Autodesk Fusion 360 part; units mm, degrees
(part 2 of 2)
  line L726 (5.1001, -37.5652) -> (5.1001, -35.2552)
  line L727 (5.1001, -35.2552) -> (3.0996, -34.1002)
  line L728 (3.0996, -25.0042) -> (1.099, -26.1592)
  line L729 (1.099, -26.1592) -> (1.099, -28.4692)
  line L730 (1.099, -28.4692) -> (3.0996, -29.6242)
  line L731 (3.0996, -29.6242) -> (5.1001, -28.4692)
  line L732 (5.1001, -28.4692) -> (5.1001, -26.1592)
  line L733 (5.1001, -26.1592) -> (3.0996, -25.0042)
  line L734 (-2.0204, -34.1002) -> (-4.021, -35.2552)
  line L735 (-4.021, -35.2552) -> (-4.021, -37.5652)
  line L736 (-4.021, -37.5652) -> (-2.0204, -38.7202)
  line L737 (-2.0204, -38.7202) -> (-0.0199, -37.5652)
  line L738 (-0.0199, -37.5652) -> (-0.0199, -35.2552)
  line L739 (-0.0199, -35.2552) -> (-2.0204, -34.1002)
  line L740 (-2.0204, -25.0042) -> (-4.021, -26.1592)
  line L741 (-4.021, -26.1592) -> (-4.021, -28.4692)
  line L742 (-4.021, -28.4692) -> (-2.0204, -29.6242)
  line L743 (-2.0204, -29.6242) -> (-0.0199, -28.4692)
  line L744 (-0.0199, -28.4692) -> (-0.0199, -26.1592)
  line L745 (-0.0199, -26.1592) -> (-2.0204, -25.0042)
  line L746 (-7.1404, -34.1002) -> (-9.141, -35.2552)
  line L747 (-9.141, -35.2552) -> (-9.141, -37.5652)
  line L748 (-9.141, -37.5652) -> (-7.1404, -38.7202)
  line L749 (-7.1404, -38.7202) -> (-5.1399, -37.5652)
  line L750 (-5.1399, -37.5652) -> (-5.1399, -35.2552)
  line L751 (-5.1399, -35.2552) -> (-7.1404, -34.1002)
  line L752 (-7.1404, -25.0042) -> (-9.141, -26.1592)
  line L753 (-9.141, -26.1592) -> (-9.141, -28.4692)
  line L754 (-9.141, -28.4692) -> (-7.1404, -29.6242)
  line L755 (-7.1404, -29.6242) -> (-5.1399, -28.4692)
  line L756 (-5.1399, -28.4692) -> (-5.1399, -26.1592)
  line L757 (-5.1399, -26.1592) -> (-7.1404, -25.0042)
  line L758 (-12.2604, -34.1002) -> (-14.261, -35.2552)
  line L759 (-14.261, -35.2552) -> (-14.261, -37.5652)
  line L760 (-14.261, -37.5652) -> (-12.2604, -38.7202)
  line L761 (-12.2604, -38.7202) -> (-10.2599, -37.5652)
  line L762 (-10.2599, -37.5652) -> (-10.2599, -35.2552)
  line L763 (-10.2599, -35.2552) -> (-12.2604, -34.1002)
  line L764 (-12.2604, -25.0042) -> (-14.261, -26.1592)
  line L765 (-14.261, -26.1592) -> (-14.261, -28.4692)
  line L766 (-14.261, -28.4692) -> (-12.2604, -29.6242)
  line L767 (-12.2604, -29.6242) -> (-10.2599, -28.4692)
  line L768 (-10.2599, -28.4692) -> (-10.2599, -26.1592)
  line L769 (-10.2599, -26.1592) -> (-12.2604, -25.0042)
  line L770 (-17.3804, -34.1002) -> (-19.381, -35.2552)
  line L771 (-19.381, -35.2552) -> (-19.381, -37.5652)
  line L772 (-19.381, -37.5652) -> (-17.3804, -38.7202)
  line L773 (-17.3804, -38.7202) -> (-15.3799, -37.5652)
  line L774 (-15.3799, -37.5652) -> (-15.3799, -35.2552)
  line L775 (-15.3799, -35.2552) -> (-17.3804, -34.1002)
  line L776 (-17.3804, -25.0042) -> (-19.381, -26.1592)
  line L777 (-19.381, -26.1592) -> (-19.381, -28.4692)
  line L778 (-19.381, -28.4692) -> (-17.3804, -29.6242)
  line L779 (-17.3804, -29.6242) -> (-15.3799, -28.4692)
  line L780 (-15.3799, -28.4692) -> (-15.3799, -26.1592)
  line L781 (-15.3799, -26.1592) -> (-17.3804, -25.0042)
  line L782 (13.8344, 32.9648) -> (13.8344, 30.6548)
  line L783 (13.8344, 30.6548) -> (15.8349, 29.4998)
  line L784 (15.8349, 29.4998) -> (17.8354, 30.6548)
  line L785 (17.8354, 30.6548) -> (17.8354, 32.9648)
  line L786 (17.8354, 32.9648) -> (15.8349, 34.1198)
  line L787 (15.8349, 34.1198) -> (13.8344, 32.9648)
  line L788 (17.8354, 23.8688) -> (15.8349, 25.0238)
  line L789 (15.8349, 25.0238) -> (13.8344, 23.8688)
  line L790 (13.8344, 23.8688) -> (13.8344, 21.5588)
  line L791 (13.8344, 21.5588) -> (15.8349, 20.4038)
  line L792 (15.8349, 20.4038) -> (17.8354, 21.5588)
  line L793 (17.8354, 21.5588) -> (17.8354, 23.8688)
  line L794 (17.8354, 14.7728) -> (15.8349, 15.9278)
  line L795 (15.8349, 15.9278) -> (13.8344, 14.7728)
  line L796 (13.8344, 14.7728) -> (13.8344, 12.4628)
  line L797 (13.8344, 12.4628) -> (15.8349, 11.3078)
  line L798 (15.8349, 11.3078) -> (17.8354, 12.4628)
  line L799 (17.8354, 12.4628) -> (17.8354, 14.7728)
  line L800 (17.8354, 5.6768) -> (15.8349, 6.8318)
  line L801 (15.8349, 6.8318) -> (13.8344, 5.6768)
  line L802 (13.8344, 5.6768) -> (13.8344, 3.3668)
  line L803 (13.8344, 3.3668) -> (15.8349, 2.2118)
  line L804 (15.8349, 2.2118) -> (17.8354, 3.3668)
  line L805 (17.8354, 3.3668) -> (17.8354, 5.6768)
  line L806 (17.8354, -3.4192) -> (15.8349, -2.2642)
  line L807 (15.8349, -2.2642) -> (13.8344, -3.4192)
  line L808 (13.8344, -3.4192) -> (13.8344, -5.7292)
  line L809 (13.8344, -5.7292) -> (15.8349, -6.8842)
  line L810 (15.8349, -6.8842) -> (17.8354, -5.7292)
  line L811 (17.8354, -5.7292) -> (17.8354, -3.4192)
  line L812 (17.8354, -12.5152) -> (15.8349, -11.3602)
  line L813 (15.8349, -11.3602) -> (13.8344, -12.5152)
  line L814 (13.8344, -12.5152) -> (13.8344, -14.8252)
  line L815 (13.8344, -14.8252) -> (15.8349, -15.9802)
  line L816 (15.8349, -15.9802) -> (17.8354, -14.8252)
  line L817 (17.8354, -14.8252) -> (17.8354, -12.5152)
  line L818 (17.8354, -21.6112) -> (15.8349, -20.4562)
  line L819 (15.8349, -20.4562) -> (13.8344, -21.6112)
  line L820 (13.8344, -21.6112) -> (13.8344, -23.9212)
  line L821 (13.8344, -23.9212) -> (15.8349, -25.0762)
  line L822 (15.8349, -25.0762) -> (17.8354, -23.9212)
  line L823 (17.8354, -23.9212) -> (17.8354, -21.6112)
  line L824 (17.8354, -30.7072) -> (15.8349, -29.5522)
  line L825 (15.8349, -29.5522) -> (13.8344, -30.7072)
  line L826 (13.8344, -30.7072) -> (13.8344, -33.0172)
  line L827 (13.8344, -33.0172) -> (15.8349, -34.1722)
  line L828 (15.8349, -34.1722) -> (17.8354, -33.0172)
  line L829 (17.8354, -33.0172) -> (17.8354, -30.7072)
  line L830 (12.7154, 32.9648) -> (10.7149, 34.1198)
  line L831 (10.7149, 34.1198) -> (8.7144, 32.9648)
  line L832 (8.7144, 32.9648) -> (8.7144, 30.6548)
  line L833 (8.7144, 30.6548) -> (10.7149, 29.4998)
  line L834 (10.7149, 29.4998) -> (12.7154, 30.6548)
  line L835 (12.7154, 30.6548) -> (12.7154, 32.9648)
  line L836 (7.5954, 32.9648) -> (5.5949, 34.1198)
  line L837 (5.5949, 34.1198) -> (3.5944, 32.9648)
  line L838 (3.5944, 32.9648) -> (3.5944, 30.6548)
  line L839 (3.5944, 30.6548) -> (5.5949, 29.4998)
  line L840 (5.5949, 29.4998) -> (7.5954, 30.6548)
  line L841 (7.5954, 30.6548) -> (7.5954, 32.9648)
  line L842 (2.4754, 32.9648) -> (0.4749, 34.1198)
  line L843 (0.4749, 34.1198) -> (-1.5256, 32.9648)
  line L844 (-1.5256, 32.9648) -> (-1.5256, 30.6548)
  line L845 (-1.5256, 30.6548) -> (0.4749, 29.4998)
  line L846 (0.4749, 29.4998) -> (2.4754, 30.6548)
  line L847 (2.4754, 30.6548) -> (2.4754, 32.9648)
  line L848 (-2.6446, 32.9648) -> (-4.6451, 34.1198)
  line L849 (-4.6451, 34.1198) -> (-6.6456, 32.9648)
  line L850 (-6.6456, 32.9648) -> (-6.6456, 30.6548)
  line L851 (-6.6456, 30.6548) -> (-4.6451, 29.4998)
  line L852 (-4.6451, 29.4998) -> (-2.6446, 30.6548)
  line L853 (-2.6446, 30.6548) -> (-2.6446, 32.9648)
  line L854 (-7.7646, 32.9648) -> (-9.7651, 34.1198)
  line L855 (-9.7651, 34.1198) -> (-11.7656, 32.9648)
  line L856 (-11.7656, 32.9648) -> (-11.7656, 30.6548)
  line L857 (-11.7656, 30.6548) -> (-9.7651, 29.4998)
  line L858 (-9.7651, 29.4998) -> (-7.7646, 30.6548)
  line L859 (-7.7646, 30.6548) -> (-7.7646, 32.9648)
  line L860 (-12.8846, 32.9648) -> (-14.8851, 34.1198)
  line L861 (-14.8851, 34.1198) -> (-16.8856, 32.9648)
  line L862 (-16.8856, 32.9648) -> (-16.8856, 30.6548)
  line L863 (-16.8856, 30.6548) -> (-14.8851, 29.4998)
  line L864 (-14.8851, 29.4998) -> (-12.8846, 30.6548)
  line L865 (-12.8846, 30.6548) -> (-12.8846, 32.9648)
  line L866 (12.7154, 23.8688) -> (10.7149, 25.0238)
  line L867 (10.7149, 25.0238) -> (8.7144, 23.8688)
  line L868 (8.7144, 23.8688) -> (8.7144, 21.5588)
  line L869 (8.7144, 21.5588) -> (10.7149, 20.4038)
  line L870 (10.7149, 20.4038) -> (12.7154, 21.5588)
  line L871 (12.7154, 21.5588) -> (12.7154, 23.8688)
  line L872 (7.5954, 23.8688) -> (5.5949, 25.0238)
  line L873 (5.5949, 25.0238) -> (3.5944, 23.8688)
  line L874 (3.5944, 23.8688) -> (3.5944, 21.5588)
  line L875 (3.5944, 21.5588) -> (5.5949, 20.4038)
  line L876 (5.5949, 20.4038) -> (7.5954, 21.5588)
  line L877 (7.5954, 21.5588) -> (7.5954, 23.8688)
  line L878 (2.4754, 23.8688) -> (0.4749, 25.0238)
  line L879 (0.4749, 25.0238) -> (-1.5256, 23.8688)
  line L880 (-1.5256, 23.8688) -> (-1.5256, 21.5588)
  line L881 (-1.5256, 21.5588) -> (0.4749, 20.4038)
  line L882 (0.4749, 20.4038) -> (2.4754, 21.5588)
  line L883 (2.4754, 21.5588) -> (2.4754, 23.8688)
  line L884 (-2.6446, 23.8688) -> (-4.6451, 25.0238)
  line L885 (-4.6451, 25.0238) -> (-6.6456, 23.8688)
  line L886 (-6.6456, 23.8688) -> (-6.6456, 21.5588)
  line L887 (-6.6456, 21.5588) -> (-4.6451, 20.4038)
  line L888 (-4.6451, 20.4038) -> (-2.6446, 21.5588)
  line L889 (-2.6446, 21.5588) -> (-2.6446, 23.8688)
  line L890 (-7.7646, 23.8688) -> (-9.7651, 25.0238)
  line L891 (-9.7651, 25.0238) -> (-11.7656, 23.8688)
  line L892 (-11.7656, 23.8688) -> (-11.7656, 21.5588)
  line L893 (-11.7656, 21.5588) -> (-9.7651, 20.4038)
  line L894 (-9.7651, 20.4038) -> (-7.7646, 21.5588)
  line L895 (-7.7646, 21.5588) -> (-7.7646, 23.8688)
  line L896 (-12.8846, 23.8688) -> (-14.8851, 25.0238)
  line L897 (-14.8851, 25.0238) -> (-16.8856, 23.8688)
  line L898 (-16.8856, 23.8688) -> (-16.8856, 21.5588)
  line L899 (-16.8856, 21.5588) -> (-14.8851, 20.4038)
  line L900 (-14.8851, 20.4038) -> (-12.8846, 21.5588)
  line L901 (-12.8846, 21.5588) -> (-12.8846, 23.8688)
  line L902 (12.7154, 14.7728) -> (10.7149, 15.9278)
  line L903 (10.7149, 15.9278) -> (8.7144, 14.7728)
  line L904 (8.7144, 14.7728) -> (8.7144, 12.4628)
  line L905 (8.7144, 12.4628) -> (10.7149, 11.3078)
  line L906 (10.7149, 11.3078) -> (12.7154, 12.4628)
  line L907 (12.7154, 12.4628) -> (12.7154, 14.7728)
  line L908 (7.5954, 14.7728) -> (5.5949, 15.9278)
  line L909 (5.5949, 15.9278) -> (3.5944, 14.7728)
  line L910 (3.5944, 14.7728) -> (3.5944, 12.4628)
  line L911 (3.5944, 12.4628) -> (5.5949, 11.3078)
  line L912 (5.5949, 11.3078) -> (7.5954, 12.4628)
  line L913 (7.5954, 12.4628) -> (7.5954, 14.7728)
  line L914 (2.4754, 14.7728) -> (0.4749, 15.9278)
  line L915 (0.4749, 15.9278) -> (-1.5256, 14.7728)
  line L916 (-1.5256, 14.7728) -> (-1.5256, 12.4628)
  line L917 (-1.5256, 12.4628) -> (0.4749, 11.3078)
  line L918 (0.4749, 11.3078) -> (2.4754, 12.4628)
  line L919 (2.4754, 12.4628) -> (2.4754, 14.7728)
  line L920 (-2.6446, 14.7728) -> (-4.6451, 15.9278)
  line L921 (-4.6451, 15.9278) -> (-6.6456, 14.7728)
  line L922 (-6.6456, 14.7728) -> (-6.6456, 12.4628)
  line L923 (-6.6456, 12.4628) -> (-4.6451, 11.3078)
  line L924 (-4.6451, 11.3078) -> (-2.6446, 12.4628)
  line L925 (-2.6446, 12.4628) -> (-2.6446, 14.7728)
  line L926 (-7.7646, 14.7728) -> (-9.7651, 15.9278)
  line L927 (-9.7651, 15.9278) -> (-11.7656, 14.7728)
  line L928 (-11.7656, 14.7728) -> (-11.7656, 12.4628)
  line L929 (-11.7656, 12.4628) -> (-9.7651, 11.3078)
  line L930 (-9.7651, 11.3078) -> (-7.7646, 12.4628)
  line L931 (-7.7646, 12.4628) -> (-7.7646, 14.7728)
  line L932 (-12.8846, 14.7728) -> (-14.8851, 15.9278)
  line L933 (-14.8851, 15.9278) -> (-16.8856, 14.7728)
  line L934 (-16.8856, 14.7728) -> (-16.8856, 12.4628)
  line L935 (-16.8856, 12.4628) -> (-14.8851, 11.3078)
  line L936 (-14.8851, 11.3078) -> (-12.8846, 12.4628)
  line L937 (-12.8846, 12.4628) -> (-12.8846, 14.7728)
  line L938 (12.7154, 5.6768) -> (10.7149, 6.8318)
  line L939 (10.7149, 6.8318) -> (8.7144, 5.6768)
  line L940 (8.7144, 5.6768) -> (8.7144, 3.3668)
  line L941 (8.7144, 3.3668) -> (10.7149, 2.2118)
  line L942 (10.7149, 2.2118) -> (12.7154, 3.3668)
  line L943 (12.7154, 3.3668) -> (12.7154, 5.6768)
  line L944 (7.5954, 5.6768) -> (5.5949, 6.8318)
  line L945 (5.5949, 6.8318) -> (3.5944, 5.6768)
  line L946 (3.5944, 5.6768) -> (3.5944, 3.3668)
  line L947 (3.5944, 3.3668) -> (5.5949, 2.2118)
  line L948 (5.5949, 2.2118) -> (7.5954, 3.3668)
  line L949 (7.5954, 3.3668) -> (7.5954, 5.6768)
  line L950 (2.4754, 5.6768) -> (0.4749, 6.8318)
  line L951 (0.4749, 6.8318) -> (-1.5256, 5.6768)
  line L952 (-1.5256, 5.6768) -> (-1.5256, 3.3668)
  line L953 (-1.5256, 3.3668) -> (0.4749, 2.2118)
  line L954 (0.4749, 2.2118) -> (2.4754, 3.3668)
  line L955 (2.4754, 3.3668) -> (2.4754, 5.6768)
  line L956 (-2.6446, 5.6768) -> (-4.6451, 6.8318)
  line L957 (-4.6451, 6.8318) -> (-6.6456, 5.6768)
  line L958 (-6.6456, 5.6768) -> (-6.6456, 3.3668)
  line L959 (-6.6456, 3.3668) -> (-4.6451, 2.2118)
  line L960 (-4.6451, 2.2118) -> (-2.6446, 3.3668)
  line L961 (-2.6446, 3.3668) -> (-2.6446, 5.6768)
  line L962 (-7.7646, 5.6768) -> (-9.7651, 6.8318)
  line L963 (-9.7651, 6.8318) -> (-11.7656, 5.6768)
  line L964 (-11.7656, 5.6768) -> (-11.7656, 3.3668)
  line L965 (-11.7656, 3.3668) -> (-9.7651, 2.2118)
  line L966 (-9.7651, 2.2118) -> (-7.7646, 3.3668)
  line L967 (-7.7646, 3.3668) -> (-7.7646, 5.6768)
  line L968 (-12.8846, 5.6768) -> (-14.8851, 6.8318)
  line L969 (-14.8851, 6.8318) -> (-16.8856, 5.6768)
  line L970 (-16.8856, 5.6768) -> (-16.8856, 3.3668)
  line L971 (-16.8856, 3.3668) -> (-14.8851, 2.2118)
  line L972 (-14.8851, 2.2118) -> (-12.8846, 3.3668)
  line L973 (-12.8846, 3.3668) -> (-12.8846, 5.6768)
  line L974 (12.7154, -3.4192) -> (10.7149, -2.2642)
  line L975 (10.7149, -2.2642) -> (8.7144, -3.4192)
  line L976 (8.7144, -3.4192) -> (8.7144, -5.7292)
  line L977 (8.7144, -5.7292) -> (10.7149, -6.8842)
  line L978 (10.7149, -6.8842) -> (12.7154, -5.7292)
  line L979 (12.7154, -5.7292) -> (12.7154, -3.4192)
  line L980 (7.5954, -3.4192) -> (5.5949, -2.2642)
  line L981 (5.5949, -2.2642) -> (3.5944, -3.4192)
  line L982 (3.5944, -3.4192) -> (3.5944, -5.7292)
  line L983 (3.5944, -5.7292) -> (5.5949, -6.8842)
  line L984 (5.5949, -6.8842) -> (7.5954, -5.7292)
  line L985 (7.5954, -5.7292) -> (7.5954, -3.4192)
  line L986 (2.4754, -3.4192) -> (0.4749, -2.2642)
  line L987 (0.4749, -2.2642) -> (-1.5256, -3.4192)
  line L988 (-1.5256, -3.4192) -> (-1.5256, -5.7292)
  line L989 (-1.5256, -5.7292) -> (0.4749, -6.8842)
  line L990 (0.4749, -6.8842) -> (2.4754, -5.7292)
  line L991 (2.4754, -5.7292) -> (2.4754, -3.4192)
  line L992 (-2.6446, -3.4192) -> (-4.6451, -2.2642)
  line L993 (-4.6451, -2.2642) -> (-6.6456, -3.4192)
  line L994 (-6.6456, -3.4192) -> (-6.6456, -5.7292)
  line L995 (-6.6456, -5.7292) -> (-4.6451, -6.8842)
  line L996 (-4.6451, -6.8842) -> (-2.6446, -5.7292)
  line L997 (-2.6446, -5.7292) -> (-2.6446, -3.4192)
  line L998 (-7.7646, -3.4192) -> (-9.7651, -2.2642)
  line L999 (-9.7651, -2.2642) -> (-11.7656, -3.4192)
  line L1000 (-11.7656, -3.4192) -> (-11.7656, -5.7292)
  line L1001 (-11.7656, -5.7292) -> (-9.7651, -6.8842)
  line L1002 (-9.7651, -6.8842) -> (-7.7646, -5.7292)
  line L1003 (-7.7646, -5.7292) -> (-7.7646, -3.4192)
  line L1004 (-12.8846, -3.4192) -> (-14.8851, -2.2642)
  line L1005 (-14.8851, -2.2642) -> (-16.8856, -3.4192)
  line L1006 (-16.8856, -3.4192) -> (-16.8856, -5.7292)
  line L1007 (-16.8856, -5.7292) -> (-14.8851, -6.8842)
  line L1008 (-14.8851, -6.8842) -> (-12.8846, -5.7292)
  line L1009 (-12.8846, -5.7292) -> (-12.8846, -3.4192)
  line L1010 (12.7154, -12.5152) -> (10.7149, -11.3602)
  line L1011 (10.7149, -11.3602) -> (8.7144, -12.5152)
  line L1012 (8.7144, -12.5152) -> (8.7144, -14.8252)
  line L1013 (8.7144, -14.8252) -> (10.7149, -15.9802)
  line L1014 (10.7149, -15.9802) -> (12.7154, -14.8252)
  line L1015 (12.7154, -14.8252) -> (12.7154, -12.5152)
  line L1016 (7.5954, -12.5152) -> (5.5949, -11.3602)
  line L1017 (5.5949, -11.3602) -> (3.5944, -12.5152)
  line L1018 (3.5944, -12.5152) -> (3.5944, -14.8252)
  line L1019 (3.5944, -14.8252) -> (5.5949, -15.9802)
  line L1020 (5.5949, -15.9802) -> (7.5954, -14.8252)
  line L1021 (7.5954, -14.8252) -> (7.5954, -12.5152)
  line L1022 (2.4754, -12.5152) -> (0.4749, -11.3602)
  line L1023 (0.4749, -11.3602) -> (-1.5256, -12.5152)
  line L1024 (-1.5256, -12.5152) -> (-1.5256, -14.8252)
  line L1025 (-1.5256, -14.8252) -> (0.4749, -15.9802)
  line L1026 (0.4749, -15.9802) -> (2.4754, -14.8252)
  line L1027 (2.4754, -14.8252) -> (2.4754, -12.5152)
  line L1028 (-2.6446, -12.5152) -> (-4.6451, -11.3602)
  line L1029 (-4.6451, -11.3602) -> (-6.6456, -12.5152)
  line L1030 (-6.6456, -12.5152) -> (-6.6456, -14.8252)
  line L1031 (-6.6456, -14.8252) -> (-4.6451, -15.9802)
  line L1032 (-4.6451, -15.9802) -> (-2.6446, -14.8252)
  line L1033 (-2.6446, -14.8252) -> (-2.6446, -12.5152)
  line L1034 (-7.7646, -12.5152) -> (-9.7651, -11.3602)
  line L1035 (-9.7651, -11.3602) -> (-11.7656, -12.5152)
  line L1036 (-11.7656, -12.5152) -> (-11.7656, -14.8252)
  line L1037 (-11.7656, -14.8252) -> (-9.7651, -15.9802)
  line L1038 (-9.7651, -15.9802) -> (-7.7646, -14.8252)
  line L1039 (-7.7646, -14.8252) -> (-7.7646, -12.5152)
  line L1040 (-12.8846, -12.5152) -> (-14.8851, -11.3602)
  line L1041 (-14.8851, -11.3602) -> (-16.8856, -12.5152)
  line L1042 (-16.8856, -12.5152) -> (-16.8856, -14.8252)
  line L1043 (-16.8856, -14.8252) -> (-14.8851, -15.9802)
  line L1044 (-14.8851, -15.9802) -> (-12.8846, -14.8252)
  line L1045 (-12.8846, -14.8252) -> (-12.8846, -12.5152)
  line L1046 (12.7154, -21.6112) -> (10.7149, -20.4562)
  line L1047 (10.7149, -20.4562) -> (8.7144, -21.6112)
  line L1048 (8.7144, -21.6112) -> (8.7144, -23.9212)
  line L1049 (8.7144, -23.9212) -> (10.7149, -25.0762)
  line L1050 (10.7149, -25.0762) -> (12.7154, -23.9212)
  line L1051 (12.7154, -23.9212) -> (12.7154, -21.6112)
  line L1052 (7.5954, -21.6112) -> (5.5949, -20.4562)
  line L1053 (5.5949, -20.4562) -> (3.5944, -21.6112)
  line L1054 (3.5944, -21.6112) -> (3.5944, -23.9212)
  line L1055 (3.5944, -23.9212) -> (5.5949, -25.0762)
  line L1056 (5.5949, -25.0762) -> (7.5954, -23.9212)
  line L1057 (7.5954, -23.9212) -> (7.5954, -21.6112)
  line L1058 (2.4754, -21.6112) -> (0.4749, -20.4562)
  line L1059 (0.4749, -20.4562) -> (-1.5256, -21.6112)
  line L1060 (-1.5256, -21.6112) -> (-1.5256, -23.9212)
  line L1061 (-1.5256, -23.9212) -> (0.4749, -25.0762)
  line L1062 (0.4749, -25.0762) -> (2.4754, -23.9212)
  line L1063 (2.4754, -23.9212) -> (2.4754, -21.6112)
  line L1064 (-2.6446, -21.6112) -> (-4.6451, -20.4562)
  line L1065 (-4.6451, -20.4562) -> (-6.6456, -21.6112)
  line L1066 (-6.6456, -21.6112) -> (-6.6456, -23.9212)
  line L1067 (-6.6456, -23.9212) -> (-4.6451, -25.0762)
  line L1068 (-4.6451, -25.0762) -> (-2.6446, -23.9212)
  line L1069 (-2.6446, -23.9212) -> (-2.6446, -21.6112)
  line L1070 (-7.7646, -21.6112) -> (-9.7651, -20.4562)
  line L1071 (-9.7651, -20.4562) -> (-11.7656, -21.6112)
  line L1072 (-11.7656, -21.6112) -> (-11.7656, -23.9212)
  line L1073 (-11.7656, -23.9212) -> (-9.7651, -25.0762)
  line L1074 (-9.7651, -25.0762) -> (-7.7646, -23.9212)
  line L1075 (-7.7646, -23.9212) -> (-7.7646, -21.6112)
  line L1076 (-12.8846, -21.6112) -> (-14.8851, -20.4562)
  line L1077 (-14.8851, -20.4562) -> (-16.8856, -21.6112)
  line L1078 (-16.8856, -21.6112) -> (-16.8856, -23.9212)
  line L1079 (-16.8856, -23.9212) -> (-14.8851, -25.0762)
  line L1080 (-14.8851, -25.0762) -> (-12.8846, -23.9212)
  line L1081 (-12.8846, -23.9212) -> (-12.8846, -21.6112)
  line L1082 (12.7154, -30.7072) -> (10.7149, -29.5522)
  line L1083 (10.7149, -29.5522) -> (8.7144, -30.7072)
  line L1084 (8.7144, -30.7072) -> (8.7144, -33.0172)
  line L1085 (8.7144, -33.0172) -> (10.7149, -34.1722)
  line L1086 (10.7149, -34.1722) -> (12.7154, -33.0172)
  line L1087 (12.7154, -33.0172) -> (12.7154, -30.7072)
  line L1088 (7.5954, -30.7072) -> (5.5949, -29.5522)
  line L1089 (5.5949, -29.5522) -> (3.5944, -30.7072)
  line L1090 (3.5944, -30.7072) -> (3.5944, -33.0172)
  line L1091 (3.5944, -33.0172) -> (5.5949, -34.1722)
  line L1092 (5.5949, -34.1722) -> (7.5954, -33.0172)
  line L1093 (7.5954, -33.0172) -> (7.5954, -30.7072)
  line L1094 (2.4754, -30.7072) -> (0.4749, -29.5522)
  line L1095 (0.4749, -29.5522) -> (-1.5256, -30.7072)
  line L1096 (-1.5256, -30.7072) -> (-1.5256, -33.0172)
  line L1097 (-1.5256, -33.0172) -> (0.4749, -34.1722)
  line L1098 (0.4749, -34.1722) -> (2.4754, -33.0172)
  line L1099 (2.4754, -33.0172) -> (2.4754, -30.7072)
  line L1100 (-2.6446, -30.7072) -> (-4.6451, -29.5522)
  line L1101 (-4.6451, -29.5522) -> (-6.6456, -30.7072)
  line L1102 (-6.6456, -30.7072) -> (-6.6456, -33.0172)
  line L1103 (-6.6456, -33.0172) -> (-4.6451, -34.1722)
  line L1104 (-4.6451, -34.1722) -> (-2.6446, -33.0172)
  line L1105 (-2.6446, -33.0172) -> (-2.6446, -30.7072)
  line L1106 (-7.7646, -30.7072) -> (-9.7651, -29.5522)
  line L1107 (-9.7651, -29.5522) -> (-11.7656, -30.7072)
  line L1108 (-11.7656, -30.7072) -> (-11.7656, -33.0172)
  line L1109 (-11.7656, -33.0172) -> (-9.7651, -34.1722)
  line L1110 (-9.7651, -34.1722) -> (-7.7646, -33.0172)
  line L1111 (-7.7646, -33.0172) -> (-7.7646, -30.7072)
  line L1112 (-12.8846, -30.7072) -> (-14.8851, -29.5522)
  line L1113 (-14.8851, -29.5522) -> (-16.8856, -30.7072)
  line L1114 (-16.8856, -30.7072) -> (-16.8856, -33.0172)
  line L1115 (-16.8856, -33.0172) -> (-14.8851, -34.1722)
  line L1116 (-14.8851, -34.1722) -> (-12.8846, -33.0172)
  line L1117 (-12.8846, -33.0172) -> (-12.8846, -30.7072)
  line L1118 (2.599, 31.0228) -> (-2.601, 31.0228)
  line L1119 (3.299, 31.7228) -> (-3.301, 31.7228)
  line L1120 (2.599, 31.0228) -> (2.599, 20.7728)
  line L1121 (3.299, 20.0728) -> (3.299, 31.7228)
  line L1122 (-0.001, 20.7728) -> (-0.001, 23.4228)
  line L1123 (2.599, 20.7728) -> (-0.001, 20.7728)
  line L1124 (-2.601, 23.4228) -> (-0.001, 23.4228)
  line L1125 (-2.601, 31.0228) -> (-2.601, 23.4228)
  line L1126 (-3.301, 31.7228) -> (-3.301, 22.7228)
  line L1127 (-3.301, 22.7228) -> (-0.701, 22.7228)
  line L1128 (-0.701, 22.7228) -> (-0.701, 20.0728)
  line L1129 (-0.701, 20.0728) -> (3.299, 20.0728)
  arc A0 (4.599, 31.0228) -> (2.599, 33.0228) centre (2.599, 31.0228) ccw
  line L1130 (4.599, 31.0228) -> (4.599, 20.7728)
  arc A1 (2.599, 18.7728) -> (4.599, 20.7728) centre (2.599, 20.7728) ccw
  line L1131 (2.599, 18.7728) -> (-0.001, 18.7728)
  arc A2 (-2.001, 20.7728) -> (-0.001, 18.7728) centre (-0.001, 20.7728) ccw
  line L1132 (-2.001, 21.4228) -> (-2.001, 20.7728)
  line L1133 (-2.001, 21.4228) -> (-2.601, 21.4228)
  arc A3 (-4.601, 23.4228) -> (-2.601, 21.4228) centre (-2.601, 23.4228) ccw
  line L1134 (-4.601, 31.0228) -> (-4.601, 23.4228)
  arc A4 (-2.601, 33.0228) -> (-4.601, 31.0228) centre (-2.601, 31.0228) ccw
  line L1135 (2.599, 33.0228) -> (-2.601, 33.0228)
  point P0 (18.4596, 36.3578)
  point P1 (16.459, 36.0228)
  point P2 (18.4596, 36.3578)
  point P3 (18.4596, 27.2618)
  point P4 (17.209, 34.7698)
  point P5 (17.209, 28.8498)
  point P6 (17.209, 26.9268)
  point P7 (19.209, 29.1368)
  point P8 (18.4596, 27.2618)
  point P9 (18.4596, 27.2618)
  point P10 (17.209, 25.6738)
  point P11 (16.459, 26.9268)
  point P12 (15.8349, 31.8098)
  dimension "d78" = 2.21
  dimension "d79" = 2.21
  dimension "d80" = 2
  dimension "d81" = 2
  dimension "d82" = 2.31
  dimension "d83" = 0.82
  dimension "d84" = 0.75
  dimension "d85" = 2.31
  dimension "d86" = 0.75
  dimension "d87" = 5.92
  dimension "d94" = -5.12
  dimension "d95" = -9.096
  dimension "d96" = 2.31
  dimension "d97" = 1.25
  dimension "d98" = 1.25
  dimension "d101" = -5.12
  dimension "d102" = -9.096
  dimension "d104" = 2
  dimension "d105" = 2
  dimension "d106" = 2
  dimension "d107" = 2
  dimension "d108" = 2
  dimension "d109" = 5
  dimension "d110" = 0.7
  dimension "d111" = 0.7
  dimension "d112" = 0.7
  dimension "d113" = 0.7
  dimension "d114" = 0.7
  dimension "d115" = 0.7
  dimension "d116" = 1.3
  dimension "d117" = 1.3
  dimension "d118" = 1.3
  dimension "d119" = 1.3
  dimension "d120" = 1.3
  dimension "d121" = 1.3
  dimension "d122" = 14.61
  dimension "d123" = 5.2
  dimension "d124" = 2.6
  dimension "d125" = 10.25
  dimension "d126" = 7.6
  constraint perpendicular L6 L10
  constraint perpendicular L11 L12
  constraint perpendicular L10 L13
  constraint vertical L14
  constraint coincident L13 P1
  constraint coincident L14 P1
  constraint vertical L20
  constraint coincident L10 P4
  constraint coincident L15 P4
  constraint coincident L10 P5
  constraint coincident L25 P5
  constraint horizontal L1135
  constraint horizontal L1133
  constraint vertical L1130
  constraint perpendicular L1130 L1131
  constraint tangent A0 L1130
  constraint tangent A1 L1131
  constraint tangent A2 L1132
  constraint tangent L1134 A4
  constraint tangent A0 L1135
  constraint tangent A4 L1135
  constraint tangent A3 L1134
  constraint tangent L1131 A2
  constraint tangent L1133 A3
  constraint tangent L1130 A1
  measures "d78" distance of L6 L11
  measures "d79" distance of L8 L13
  measures "d80" distance of L9 L12
  measures "d81" distance of L7 L10
  measures "d82" distance of L14.start L14.end
  measures "d83" distance of L14.end P1
  measures "d84" distance of L10 L14
  measures "d85" distance of L20.start L20.end
  measures "d86" distance of L10 L20
  measures "d87" distance of P4 P5
  measures "d96" distance of L782.start L782.end
  measures "d97" distance of L15 L786
  measures "d98" distance of L25 L784
  measures "d104" radius of A0
  measures "d105" radius of A1
  measures "d106" radius of A2
  measures "d107" radius of A3
  measures "d108" radius of A4
  measures "d109" distance of L13 L1118
  measures "d110" distance of L1118 L1119
  measures "d111" distance of L1120 L1121
  measures "d112" distance of L1123 L1129
  measures "d113" distance of L1122 L1128
  measures "d114" distance of L1124 L1127
  measures "d115" distance of L1125 L1126
  measures "d116" distance of L1121 L1130
  measures "d117" distance of L1119 L1135
  measures "d118" distance of L1126 L1134
  measures "d119" distance of L1127 L1133
  measures "d120" distance of L1128 L1132
  measures "d121" distance of L1129 L1131
  measures "d122" distance of L10 L1120
  measures "d123" distance of L1120 L1125
  measures "d124" distance of L1120 L1122
  measures "d125" distance of L1118 L1123
  measures "d126" distance of L1118 L1124
extrude "Extrude8" cut sketch "Sketch6" against normal through all contours L884 L885 L886 L887 L888 A3 L1134 | L95 L96 L97 L191 L192 L193 L1130 | L872 L873 L875 L876 L877 L1130 | L183 L184 L185 L186 L187 L279 L280 L281 L282 L283 A1 L1131 | L848 L849 L850 L851 L852 L1134 A4 | L836 L837 L838 L839 L840 L841 A0 L1130 | L842 L843 L1135 | L194 L195 L196 L197 L198 L199 L290 L291 L292 L293 L294 L295 A2 | L11 L12 L774 L775 | L11 L758 L759 L762 L763 | L12 L683 L684 L685 L779 L780 L781 | L11 L746 L747 L750 L751 | L12 L593 L594 L595 L689 L690 L691 | L11 L734 L735 L738 L739 | L12 L503 L504 L505 L599 L600 L601 | L11 L722 L723 L726 L727 | L12 L413 L414 L415 L509 L510 L511 | L11 L710 L711 L714 L715 | L12 L323 L324 L325 L419 L420 L421 | L11 L698 L699 L702 L703 | L12 L233 L234 L235 L329 L330 L331 | L10 L11 L62 L63 | L12 L143 L144 L145 L239 L240 L241 | L12 L13 L149 L150 | L10 L56 L57 L58 L692 L693 L694 | L10 L824 L825 L826 L827 L828 | L10 L50 L51 L52 L602 L603 L604 | L10 L818 L819 L820 L821 L822 | L13 L135 L136 L137 L138 | L10 L44 L45 L46 L512 L513 L514 | L10 L812 L813 L814 L815 L816 | L13 L123 L124 L125 L126 | L10 L38 L39 L40 L422 L423 L424 | L10 L806 L807 L808 L809 L810 | L13 L111 L112 L113 L114 | L10 L32 L33 L34 L332 L333 L334 | L10 L800 L801 L802 L803 L804 | L13 L99 L100 L101 L102 | L10 L26 L27 L28 L242 L243 L244 | L10 L794 L795 L796 L797 L798 | L13 L87 L88 L89 L90 | L10 L20 L21 L25 L152 L153 L154 | L10 L788 L789 L790 L791 L792 | L13 L75 L76 L77 L78 | L10 L13 L14 L15 | L10 L782 L783 L784 L786 L787 | L68 L69 L70 L71 L72 L73 L164 L165 L166 L167 L168 L169 | L80 L81 L82 L83 L84 L85 L176 L177 L178 L179 L180 L181 | L116 L117 L118 L119 L120 L121 L212 L213 L214 L215 L216 L217 | L128 L129 L130 L131 L132 L133 L224 L225 L226 L227 L228 L229 | L158 L159 L160 L161 L162 L163 L254 L255 L256 L257 L258 L259 | L170 L171 L172 L173 L174 L175 L266 L267 L268 L269 L270 L271 | L206 L207 L208 L209 L210 L211 L302 L303 L304 L305 L306 L307 | L218 L219 L220 L221 L222 L223 L314 L315 L316 L317 L318 L319 | L248 L249 L250 L251 L252 L253 L344 L345 L346 L347 L348 L349 | L260 L261 L262 L263 L264 L265 L356 L357 L358 L359 L360 L361 | L272 L273 L274 L275 L276 L277 L368 L369 L370 L371 L372 L373 | L284 L285 L286 L287 L288 L289 L380 L381 L382 L383 L384 L385 | L296 L297 L298 L299 L300 L301 L392 L393 L394 L395 L396 L397 | L308 L309 L310 L311 L312 L313 L404 L405 L406 L407 L408 L409 | L338 L339 L340 L341 L342 L343 L434 L435 L436 L437 L438 L439 | L350 L351 L352 L353 L354 L355 L446 L447 L448 L449 L450 L451 | L362 L363 L364 L365 L366 L367 L458 L459 L460 L461 L462 L463 | L374 L375 L376 L377 L378 L379 L470 L471 L472 L473 L474 L475 | L386 L387 L388 L389 L390 L391 L482 L483 L484 L485 L486 L487 | L398 L399 L400 L401 L402 L403 L494 L495 L496 L497 L498 L499 | L428 L429 L430 L431 L432 L433 L524 L525 L526 L527 L528 L529 | L440 L441 L442 L443 L444 L445 L536 L537 L538 L539 L540 L541 | L452 L453 L454 L455 L456 L457 L548 L549 L550 L551 L552 L553 | L464 L465 L466 L467 L468 L469 L560 L561 L562 L563 L564 L565 | L476 L477 L478 L479 L480 L481 L572 L573 L574 L575 L576 L577 | L488 L489 L490 L491 L492 L493 L584 L585 L586 L587 L588 L589 | L518 L519 L520 L521 L522 L523 L614 L615 L616 L617 L618 L619 | L530 L531 L532 L533 L534 L535 L626 L627 L628 L629 L630 L631 | L542 L543 L544 L545 L546 L547 L638 L639 L640 L641 L642 L643 | L554 L555 L556 L557 L558 L559 L650 L651 L652 L653 L654 L655 | L566 L567 L568 L569 L570 L571 L662 L663 L664 L665 L666 L667 | L578 L579 L580 L581 L582 L583 L674 L675 L676 L677 L678 L679 | L608 L609 L610 L611 L612 L613 L704 L705 L706 L707 L708 L709 | L620 L621 L622 L623 L624 L625 L716 L717 L718 L719 L720 L721 | L632 L633 L634 L635 L636 L637 L728 L729 L730 L731 L732 L733 | L644 L645 L646 L647 L648 L649 L740 L741 L742 L743 L744 L745 | L656 L657 L658 L659 L660 L661 L752 L753 L754 L755 L756 L757 | L668 L669 L670 L671 L672 L673 L764 L765 L766 L767 L768 L769 | L830 L831 L832 L833 L834 L835 | L854 L855 L856 L857 L858 L859 | L860 L861 L862 L863 L864 L865 | L866 L867 L868 L869 L870 L871 | L890 L891 L892 L893 L894 L895 | L896 L897 L898 L899 L900 L901 | L902 L903 L904 L905 L906 L907 | L908 L909 L910 L911 L912 L913 | L914 L915 L916 L917 L918 L919 | L920 L921 L922 L923 L924 L925 | L926 L927 L928 L929 L930 L931 | L932 L933 L934 L935 L936 L937 | L938 L939 L940 L941 L942 L943 | L944 L945 L946 L947 L948 L949 | L950 L951 L952 L953 L954 L955 | L956 L957 L958 L959 L960 L961 | L962 L963 L964 L965 L966 L967 | L968 L969 L970 L971 L972 L973 | L974 L975 L976 L977 L978 L979 | L980 L981 L982 L983 L984 L985 | L986 L987 L988 L989 L990 L991 | L992 L993 L994 L995 L996 L997 | L998 L999 L1000 L1001 L1002 L1003 | L1004 L1005 L1006 L1007 L1008 L1009 | L1010 L1011 L1012 L1013 L1014 L1015 | L1016 L1017 L1018 L1019 L1020 L1021 | L1022 L1023 L1024 L1025 L1026 L1027 | L1028 L1029 L1030 L1031 L1032 L1033 | L1034 L1035 L1036 L1037 L1038 L1039 | L1040 L1041 L1042 L1043 L1044 L1045 | L1046 L1047 L1048 L1049 L1050 L1051 | L1052 L1053 L1054 L1055 L1056 L1057 | L1058 L1059 L1060 L1061 L1062 L1063 | L1064 L1065 L1066 L1067 L1068 L1069 | L1070 L1071 L1072 L1073 L1074 L1075 | L1076 L1077 L1078 L1079 L1080 L1081 | L1082 L1083 L1084 L1085 L1086 L1087 | L1088 L1089 L1090 L1091 L1092 L1093 | L1094 L1095 L1096 L1097 L1098 L1099 | L1100 L1101 L1102 L1103 L1104 L1105 | L1106 L1107 L1108 L1109 L1110 L1111 | L1112 L1113 L1114 L1115 L1116 L1117
